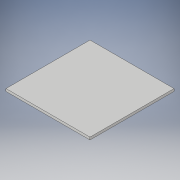
# Autodesk Inventor part: Sheet_3mm
Saved by Autodesk Inventor 2019 (Build 230136000, 136)
## iProperties
Created: 2019-09-03
Part Number: Sheet_3mm
Material: Generic
Document SubType Name: Modeling
Designer: 19879326
Density: 1 g/cm^3
Appearance: Default
Author: 19879326
Autodesk Inventor part; units mm, degrees
ref_plane "YZ Plane" through (0, 0, 0) normal (1, 0, 0) x (0, 1, 0)
ref_plane "XZ Plane" through (0, 0, 0) normal (0, 1, 0) x (-1, 0, 0)
ref_plane "XY Plane" through (0, 0, 0) normal (0, 0, 1) x (1, 0, 0)
sketch "Sketch1" plane through (0, 0, 0) normal (0, 1, 0) x (-1, 0, 0)
  line L0 (50.4, 50.4) -> (-50.4, 50.4)
  line L1 (-50.4, 50.4) -> (-50.4, -50.4)
  line L2 (-50.4, -50.4) -> (50.4, -50.4)
  line L3 (50.4, -50.4) -> (50.4, 50.4)
  point P0 (0, 0)
  point P1 (0, -50.4)
  point P2 (50.4, 0)
  dimension "d0" = 100.8
  constraints: 8 end point, 2 midpoint, 2 parallel, 2 perpendicular, 1 horizontal, 1 horizontal alignment, 1 vertical alignment
  measures "d0" distance of L2.end L0.start
extrude "Extrusion1" add sketch "Sketch1" along normal blind 3
body "Solid1"
